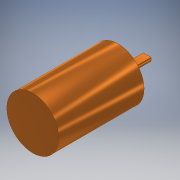
# Autodesk Inventor part: 电机
Saved by Autodesk Inventor 2018 (Build 220112000, 112)
## iProperties
Created: 2020-11-22
Part Number: 电机
Material: 金色
Document SubType Name: Modeling
Designer: OHHHHHHHHHH
Density: 19.3 g/cm^3
Appearance: 金属(1600F 火灼)
Author: OHHHHHHHHHH
Autodesk Inventor part; units mm, degrees
ref_plane "YZ Plane" through (0, 0, 0) normal (1, 0, 0) x (0, 1, 0)
ref_plane "XZ Plane" through (0, 0, 0) normal (0, 1, 0) x (-1, 0, 0)
ref_plane "XY Plane" through (0, 0, 0) normal (0, 0, 1) x (1, 0, 0)
sketch "草图1" plane through (0, 0, 0) normal (0, 1, 0) x (-1, 0, 0)
  circle A0 centre (0, 0) radius 12.5
  dimension "d0" = 25
  constraints: 1 centre point, 1 coincident
  measures "d0" diameter of A0
extrude "拉伸1" add sketch "草图1" along normal blind 41
sketch "草图2" plane through (0, 41, 0) normal (0, 1, 0) x (1, 0, 0)
  circle A0 centre (0, 0) radius 3.5
  dimension "d3" = 7
  constraints: 1 centre point, 1 coincident
  measures "d3" diameter of A0
extrude "拉伸2" add sketch "草图2" along normal blind 3
sketch "草图3" plane through (0, 44, 0) normal (0, 1, 0) x (1, 0, 0)
  circle A0 centre (0, 0) radius 2
  dimension "d6" = 4
  constraints: 1 centre point, 1 coincident
  measures "d6" diameter of A0
extrude "拉伸3" add sketch "草图3" along normal blind 11
sketch "草图4" plane through (0, 55, 0) normal (0, 1, 0) x (1, 0, 0)
  line L0 (-4.637, -0.8) -> (5.5705, -0.8)
  line L1 (-17.5, 0) -> (17.5, 0) projected
  arc A0 (-1.833, -0.8) -> (1.833, -0.8) centre (0, 0) ccw
  dimension "d9" = 0.8
  dimension "d10" = 2
  constraints: 2 end point, 2 point on circle, 2 point on line, 1 centre point, 1 coincident, 1 horizontal
  measures "d9" distance between parallel lines of L1 L0
  measures "d10" radius of A0
extrude "拉伸4" cut sketch "草图4" against normal blind 11
